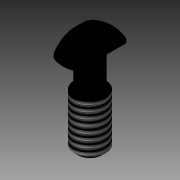
# Autodesk Inventor part: 2059_screw
Saved by Autodesk Inventor 2014 SP2 (Build 180246200, 246)
## iProperties
Created: 2018-07-19
Part Number: 2059_screw
Material: Generic
Catalog Web Link: www.cadenas.de
Description: 2059, 2051_screw-Top Mount Bi-Fold Door Hanger Assembly
Vendor: 8020
Document SubType Name: Modeling
Designer: psadmin
Manufacturer: 8020
Mass: 0.559109 g
Surface Area: 5.33056 cm^2
Volume: 0.559109 cm^3
Density: 1 g/cm^3
Appearance: PSOLRGB-0-0-0
Category: PARTsolutions
Company: 8020
Title: 2059_screw
Author: Cadenas PARTsolutions
Comments: Top Mount Bi-Fold Door Hanger Assembly
PSOL_IDENT_0: {$CADENAS_DATA\23d-libs\8020\inch\panels_and_doors\2059_screw.prj},170 {VTYP=3D},{NB=2059_screw},{LI
PSOL_IDENT_1: NA=2059_screw},{NN=2059, 2051_screw},{DATE=16.03.2018 08:23:48},{GEOMDATE=19.01.2012 13:16:00},{VERS
PSOL_IDENT_2: ION=},{LINEID=10},{WBVAR=},{WBNUMERIC=}  {NB=2059_screw},{LINA=2059_screw},{KT=DUMMY},{PN=2059},{TS=
PSOL_IDENT_3: 1/4-20 x .410},{THRD=0.2500},{L=0.410}
NN: 2059, 2051_screw
NT: Top Mount Bi-Fold Door Hanger Assembly
NB: 2059_screw
NBSYN: $PN._screw
LINA: 2059_screw
PN: 2059
TS: 1/4-20 x .410
THRD: 0.25
L: 0.41
SUPPLIER: 8020
ARTICLENO: 2059_screw
BOMINFO: 2059_screw
CREATOR: CADENAS GmbH
Autodesk Inventor part; units mm, degrees
sketch "Sketch_1" plane through (0, 0, 0) normal (0, 0, 1) x (1, 0, 0)
  line L0 (0, 0) -> (0, 20.574)
  line L1 (0, 20.574) -> (2.6561, 20.574)
  arc A0 (5.5506, 18.0111) -> (2.6561, 20.574) centre (0.9891, 15.7753) ccw
  line L2 (5.5506, 18.0111) -> (5.5506, 17.2237)
  line L3 (5.5506, 17.2237) -> (2.3752, 17.2237)
  line L4 (2.3752, 17.2237) -> (2.3752, 10.414)
  line L5 (2.3752, 10.414) -> (3.175, 10.414)
  line L6 (3.175, 10.414) -> (3.175, 0.7557)
  line L7 (3.175, 0.7557) -> (2.4194, 0)
  line L8 (2.4194, 0) -> (0, 0)
  line L9 (0, 0) -> (0, 20.574)
  constraints: 20 end point, 2 point on circle, 1 centre point
revolve "Revolution1" add sketch "Sketch_1" angle 360 about axis through (0, 0, 0) along (0, -1, 0)
thread "Thread1" size "1/4-20 UNC" class "2A" standard "ANSI Unified Screw Threads" full length
sketch "Sketch_2" plane through (0, 20.574, 0) normal (0, 1, 0) x (1, 0, 0)
  line L0 (-7.62, 7.62) -> (-7.62, -7.62)
  line L1 (-7.62, -7.62) -> (7.62, -7.62)
  line L2 (7.62, -7.62) -> (7.62, 7.62)
  line L3 (7.62, 7.62) -> (-7.62, 7.62)
  line L4 (-2.3752, 6.35) -> (-2.3752, -6.35)
  line L5 (-2.3752, -6.35) -> (2.3752, -6.35)
  line L6 (2.3752, -6.35) -> (2.3752, 6.35)
  line L7 (2.3752, 6.35) -> (-2.3752, 6.35)
  constraints: 16 end point
extrude "Extrusion1" cut sketch "Sketch_2" along normal mid plane 10.16
sketch "Sketch_3" plane through (0, 20.574, 0) normal (0, 1, 0) x (1, 0, 0)
  line L0 (-1.9814, -1.144) -> (0, -2.288)
  line L1 (0, -2.288) -> (1.9814, -1.144)
  line L2 (1.9814, -1.144) -> (1.9814, 1.144)
  line L3 (1.9814, 1.144) -> (0, 2.288)
  line L4 (0, 2.288) -> (-1.9814, 1.144)
  line L5 (-1.9814, 1.144) -> (-1.9814, -1.144)
  constraints: 12 end point
extrude "Extrusion2" cut sketch "Sketch_3" against normal blind 2.2098
ref_plane "to_a_XY" through (0, 9.6037, 0) normal (0, 1, 0) x (1, 0, 0)
ref_plane "to_a_YZ" through (0, 9.6037, 0) normal (1, 0, 0) x (0, 0, -1)
ref_plane "to_a_ZX" through (0, 9.6037, 0) normal (0, 0, -1) x (0, 1, 0)
body "Solid1"
